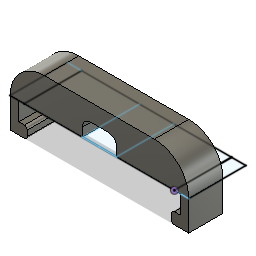
Motor Wire Cover v4 (Autodesk Fusion 360 design; units mm, degrees)
Autodesk Fusion 360 part; units mm, degrees
sketch "Sketch1" plane through (0, 0, 0) normal (0, 1, 0) x (1, 0, 0) in component "Motor Wire Cover"
  line L0 (0, 0) -> (-26.25, 0)
  line L1 (-26.25, 0) -> (-26.25, 10)
  line L2 (-26.25, 10) -> (0, 10)
  line L3 (0, 10) -> (0, 0)
  line L4 (0, 10) -> (2.5, 10)
  line L5 (2.5, 10) -> (2.5, 0)
  line L6 (2.5, 0) -> (0, 0)
  line L7 (0, 0) -> (0, 10)
  line L8 (-26.25, 0) -> (-28.75, 0)
  line L9 (-28.75, 0) -> (-28.75, 10)
  line L10 (-28.75, 10) -> (-26.25, 10)
  line L11 (-26.25, 10) -> (-26.25, 0)
  line L12 (-13.125, 0) -> (-16.125, 0)
  line L13 (-13.125, 0) -> (-10.125, 0)
  line L14 (-16.125, 0) -> (-16.125, 10)
  line L15 (-10.125, 0) -> (-10.125, 10)
  dimension "d1" = 26.25
  dimension "d2" = 10
  dimension "d3" = 2.5
  dimension "d4" = 2.5
  dimension "d5" = 3
  dimension "d6" = 3
  constraint horizontal L0
  constraint vertical L1
  constraint horizontal L2
  constraint vertical L3
  constraint coincident L0.start L3.end
  constraint midpoint L0 L12.start
  constraint horizontal L4
  constraint vertical L5
  constraint horizontal L6
  constraint vertical L7
  constraint horizontal L8
  constraint vertical L9
  constraint horizontal L10
  constraint vertical L11
  constraint coincident L2 L14.end
  constraint perpendicular L2 L14
  constraint coincident L2 L15.end
  constraint perpendicular L2 L15
  measures "d1" distance of L0.start L0.end
  measures "d2" distance of L0.start L2.end
  measures "d3" distance of L2.end L4.end
  measures "d4" distance of L0.end L8.end
  measures "d5" distance of L12.start L12.end
  measures "d6" distance of L12.start L13.end
extrude "Extrude1" add sketch "Sketch1" along normal blind 6 in component "Motor Wire Cover"
extrude "Extrude2" cut sketch "Sketch1" along normal blind 3 contours L0 L2 L12 L13 L14 L15 in component "Motor Wire Cover"
fillet "Fillet1" radius 1.5 2 edges at (-10.125, 3, -5) (-16.125, 3, -5) in component "Motor Wire Cover"
extrude "Extrude3" add sketch "Sketch1" against normal blind 3.25 contours L3 L4 L5 L6 L7 | L1 L8 L9 L10 L11 in component "Motor Wire Cover"
extrude "Extrude4" add 2 faces at (0.8333, -3.25, -6.6667) (-27.9167, -3.25, -6.6667) along direction (0, -1, 0) blind 2 in component "Motor Wire Cover"
sketch "Sketch2" plane through (0, 0, 0) normal (-1, 0, 0) x (0, 0, 1) in component "Motor Wire Cover"
  line L0 (0, 0) -> (-10, 0)
  line L1 (-10, 0) -> (-10, -5.25)
  line L2 (-10, -5.25) -> (0, -5.25)
  line L3 (0, -5.25) -> (0, 0)
  line L4 (0, -5.25) -> (-10, -5.25)
  line L5 (-10, -5.25) -> (-10, -3.25)
  line L6 (-10, -3.25) -> (0, -3.25)
  line L7 (0, -3.25) -> (0, -5.25)
  dimension "d17" = 2
  constraint horizontal L4
  constraint vertical L5
  constraint horizontal L6
  constraint vertical L7
  constraint coincident L2.end L3.start
  measures "d17" distance of L2.end L6.end
extrude "Extrude5" add sketch "Sketch2" along normal blind 2 contours L1 L2 L3 L4 L5 L6 L7 in component "Motor Wire Cover"
sketch "Sketch3" plane through (-26.25, 0, 0) normal (1, 0, 0) x (0, 0, -1) in component "Motor Wire Cover"
  line L0 (10, 0) -> (0, 0)
  line L1 (0, 0) -> (0, -5.25)
  line L2 (0, -5.25) -> (10, -5.25)
  line L3 (10, -5.25) -> (10, 0)
  line L4 (10, -5.25) -> (0, -5.25)
  line L5 (0, -5.25) -> (0, -3.25)
  line L6 (0, -3.25) -> (10, -3.25)
  line L7 (10, -3.25) -> (10, -5.25)
  dimension "d20" = 2
  constraint horizontal L4
  constraint vertical L5
  constraint horizontal L6
  constraint vertical L7
  constraint coincident L2.end L3.start
  measures "d20" distance of L2.end L6.end
extrude "Extrude6" add sketch "Sketch3" along normal blind 2 contours L1 L2 L3 L4 L5 L6 L7 in component "Motor Wire Cover"
fillet "Fillet2" radius 6 2 edges at (2.5, 6, -5) (-28.75, 6, -5) in component "Motor Wire Cover"
fillet "Fillet3" radius 1 2 edges at (-2, -3.25, -5) (-24.25, -3.25, -5) in component "Motor Wire Cover"
extrude "Extrude7" cut 3 faces at (-21.7083, 2.5, -10) (-27.9167, -2.8333, -10) (-25.25, -4.25, -10) along direction (0, 0, 1) blind 4 in component "Motor Wire Cover"
extrude "Extrude8" cut 1 faces at (0, -2.1667, -2) along direction (1, 0, 0) blind 0.5 in component "Motor Wire Cover"
extrude "Extrude9" cut 1 faces at (-26.25, -2.1667, -4) along direction (-1, 0, 0) blind 0.5 in component "Motor Wire Cover"
delete_face "DeleteFace1" 1 faces at (-1.0476, -3.2511, -4) in component "Motor Wire Cover"
delete_face "DeleteFace2" 1 faces at (-24.7918, -3.3612, -2) in component "Motor Wire Cover"
extrude "Extrude10" cut 1 faces at (-24.25, -3.9167, -2) along direction (-1, 0, 0) blind 0.5 in component "Motor Wire Cover"
extrude "Extrude11" cut 1 faces at (-2, -3.9167, -4) along direction (1, 0, 0) blind 0.5 in component "Motor Wire Cover"
extrude "Extrude12" cut 1 faces at (0.5, -2.1667, -2) along direction (1, 0, 0) blind 0.5 in component "Motor Wire Cover"
extrude "Extrude13" cut 1 faces at (-26.75, -2.1667, -4) along direction (-1, 0, 0) blind 0.5 in component "Motor Wire Cover"
extrude "Extrude14" cut 1 faces at (-1.5, -3.9167, -4) along direction (1, 0, 0) blind 0.5 in component "Motor Wire Cover"
extrude "Extrude15" cut 1 faces at (-1, -3.9167, -4) along direction (1, 0, 0) blind 0.5 in component "Motor Wire Cover"
extrude "Extrude16" cut 1 faces at (-24.75, -3.9167, -2) along direction (-1, 0, 0) blind 1 in component "Motor Wire Cover"
fillet "Fillet6" radius 0.5 4 edges at (-25.75, -3.25, -3) (-25.75, -5.25, -3) (-0.5, -5.25, -3) (-0.5, -3.25, -3) in component "Motor Wire Cover"
component "Motor Wire Cover" placed x (1, 0, 0) y (0, 1, 0) z (0, 0, 1) at (0, 0, 0)
